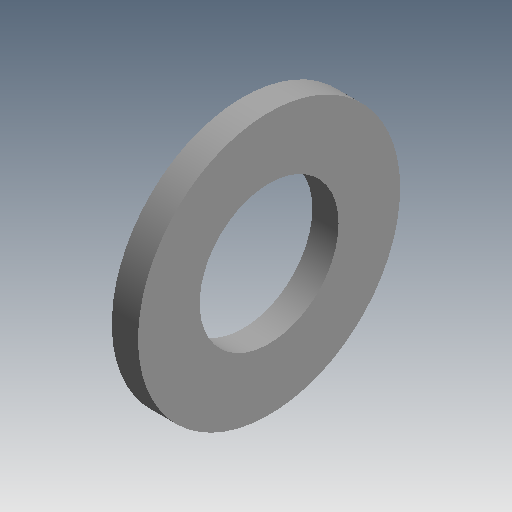
# Autodesk Inventor part: SPWF5
Saved by Autodesk Inventor 2020 (Build 240168000, 168)
## iProperties
Part Number: SPWF5
Material: Generic
Catalog Web Link: www.cadenas.de
Description: PWF, SPWF-Flat Washers
Vendor: MISUMI
Document SubType Name: Modeling
Designer: partserver
Manufacturer: MISUMI
Mass: 0.056478 g
Surface Area: 1.61022 cm^2
Volume: 0.056478 cm^3
Density: 1 g/cm^3
Appearance: PSOLRGB-192-192-192
Category: PARTsolutions
Company: MISUMI
PSOL_IDENT_0: {$CADENAS_DATA\23d-libs\misumi\metric\27_screws_nuts\pwf.prj},156 {VTYP=3D},{NB=SPWF5},{LINA=SPWF5},
PSOL_IDENT_1: {NN=PWF, SPWF},{DATE=09.09.2019 15:27:56},{GEOMDATE=15.04.2019 01:52:35},{VERSION=},{LINEID=40},{WBV
PSOL_IDENT_2: AR=MAT},{WBNUMERIC=}  {NB=SPWF5},{LINA=SPWF5},{KT=DUMMY},{PN=SPWF5},{MAT=S},{ST=Trivalent Chromate P
PSOL_IDENT_3: lating},{NO=5},{DD=5.3},{D=10.0},{D1=10.0},{D2=10.0},{TT=1.0},{M1=5.000}
NB: SPWF5
NN: PWF, SPWF
NT: Flat Washers
NBSYN: $PN.
LINA: SPWF5
CATALOG: Misumi
PN: SPWF5
MAT: 304 Stainless Steel
ST: Trivalent Chromate Plating
NO: 5
DD: 5.3
D: 10
TT: 1
SUPPLIER: MISUMI
ARTICLENO: SPWF5
BOMINFO: SPWF5
CREATOR: CADENAS GmbH
Title: SPWF5
Author: Cadenas PARTsolutions
Comments: Flat Washers
Autodesk Inventor part; units mm, degrees
sketch "Sketch_1" plane through (0, 0, 0) normal (0, 0, 1) x (1, 0, 0)
  line L0 (0.5, 0) -> (-0.5, 0)
  line L1 (-0.5, 5) -> (-0.5, 2.65)
  line L2 (-0.5, 2.65) -> (0.5, 2.65)
  line L3 (0.5, 2.65) -> (0.5, 5)
  line L4 (0.5, 5) -> (-0.5, 5)
  constraints: 10 end point
revolve "Revolution1" add sketch "Sketch_1" angle 360 about axis through (0.5, 0, 0) along (1, 0, 0)
ref_plane "plain_washer_to_bolt_XY" through (0, 0, 0) normal (1, 0, 0) x (0, 0, -1)
ref_plane "plain_washer_to_bolt_YZ" through (0, 0, 0) normal (0, 0, -1) x (0, 1, 0)
ref_plane "plain_washer_to_bolt_ZX" through (0, 0, 0) normal (0, 1, 0) x (1, 0, 0)
ref_plane "to_body_XY" through (0.5, 0, 0) normal (1, 0, 0) x (0, 0, -1)
ref_plane "to_body_YZ" through (0.5, 0, 0) normal (0, 0, -1) x (0, 1, 0)
ref_plane "to_body_ZX" through (0.5, 0, 0) normal (0, 1, 0) x (1, 0, 0)
ref_plane "to_washer_XY" through (-0.5, 0, 0) normal (1, 0, 0) x (0, 0, -1)
ref_plane "to_washer_YZ" through (-0.5, 0, 0) normal (0, 0, -1) x (0, 1, 0)
ref_plane "to_washer_ZX" through (-0.5, 0, 0) normal (0, 1, 0) x (1, 0, 0)
body "Solid1"
